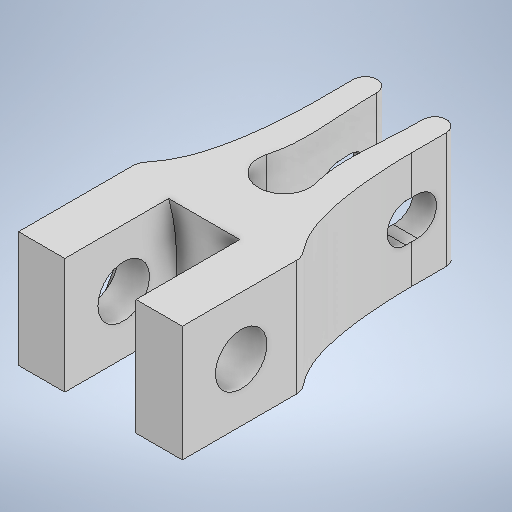
# Autodesk Inventor part: SlideClip
Saved by Autodesk Inventor 2025 (Build 290162010, 162A)
## iProperties
Created: 2025-02-04
Part Number: SlideClip
Material: Generic
Document SubType Name: Modeling
Designer: armenanzasn25
Density: 1 g/cm^3
Appearance: Default
Author: armenanzasn25
Autodesk Inventor part; units mm, degrees
ref_plane "YZ Plane" through (0, 0, 0) normal (1, 0, 0) x (0, 1, 0)
ref_plane "XZ Plane" through (0, 0, 0) normal (0, 1, 0) x (-1, 0, 0)
ref_plane "XY Plane" through (0, 0, 0) normal (0, 0, 1) x (1, 0, 0)
sketch "Sketch1" plane through (0, 0, 0) normal (0, 1, 0) x (-1, 0, 0)
  arc A0 (2.1415, -16.469) -> (0, -13.652) centre (0, -15.8745) ccw
  line L0 (7.0734, 0) -> (7.0734, -9.8745)
  line L1 (0, 0.4443) -> (0, -21.7427) construction
  line L2 (-7.0734, 0) -> (-7.0734, -9.8745)
  arc A1 (0, -13.652) -> (-2.1415, -16.469) centre (0, -15.8745) ccw
  line L3 (4, -22.8384) -> (4, -25.8745)
  line L4 (-4, -22.8384) -> (-4, -25.8745)
  arc A2 (2, -25.8745) -> (4, -25.8745) centre (3, -25.8745) ccw
  arc A3 (-4, -25.8745) -> (-2, -25.8745) centre (-3, -25.8745) ccw
  line L5 (3.0734, 0) -> (3.0734, -9.652)
  line L6 (3.0734, -9.652) -> (-3.0734, -9.652)
  line L7 (-3.0734, -9.652) -> (-3.0734, 0)
  line L8 (7.0734, 0) -> (3.0734, 0)
  line L9 (-3.0734, 0) -> (-7.0734, 0)
  spline S0 degree 4 poles (2, -25.8745) (2, -23.2445) (1.6155, -19.943) (1.6024, -18.411) (2.1415, -16.469) knots 0 0 0 0 0 1 1 1 1 1
  spline S1 degree 4 poles (-2, -25.8745) (-2, -23.2445) (-1.6155, -19.943) (-1.6024, -18.411) (-2.1415, -16.469) knots 0 0 0 0 0 1 1 1 1 1
  spline S2 degree 4 poles (7.0734, -9.8745) (7.0734, -11.5508) (4.5976, -10.8217) (4, -18.7622) (4, -22.8384) knots 0 0 0 0 0 1 1 1 1 1
  spline S3 degree 4 poles (-7.0734, -9.8745) (-7.0734, -11.5508) (-4.5976, -10.8217) (-4, -18.7622) (-4, -22.8384) knots 0 0 0 0 0 1 1 1 1 1
  point P0 (0, 0)
  point P1 (0, -9.652)
  point P2 (1.75, -19.9116)
  point P3 (-1.75, -19.9116)
  point P4 (6.2466, -11.4624)
  point P5 (-6.2466, -11.4624)
  dimension "d6" = 6
  dimension "d7" = 1
  dimension "d8" = 2.2225
  dimension "d19" = 9.652
  dimension "d20" = 6.1468
  dimension "d27" = 4
  dimension "d31" = 4
  dimension "d34" = 3.5
  dimension "d35" = 10
  dimension "d37" = 4
  constraints: 20 end point, 9 symmetric about line, 8 point on circle, 5 perpendicular, 5 vertical, 4 centre point, 2 horizontal alignment, 2 point on line, 1 collinear, 1 horizontal, 1 midpoint, 1 parallel, 1 tangent, 18 other
  measures "d6" vertical distance of L0.end A0.centre
  measures "d7" radius of A2
  measures "d8" radius of A0
  measures "d19" distance of L6.end L7.end
  measures "d20" distance of L5.end L6.end
  measures "d27" distance of point (0, -9.652) A0.end
  measures "d31" distance of L0.start L5.start
  measures "d34" distance of point (-1.75, -19.912) point (1.75, -19.912)
  measures "d35" vertical distance of A0.centre A3.centre
  measures "d37" distance of A3.end A2.start
extrude "Extrusion1" add sketch "Sketch1" along normal blind 10
sketch "Sketch2" plane through (7.0734, 0, 0) normal (1, 0, 0) x (0, 0, -1)
  circle A0 centre (5.08, 5) radius 2.2225
  line L0 (0, 10) -> (9.8745, 10) projected
  line L1 (0, 0) -> (0, 10) projected
  point P0 (9.652, 10)
  dimension "d14" = 4.445
  dimension "d15" = 5
  dimension "d32" = 4.572
  constraints: 1 centre point
  measures "d14" diameter of A0
  measures "d15" distance from line of L0 A0.centre
  measures "d32" horizontal distance of point (9.652, 10) A0.centre
extrude "Extrusion2" cut sketch "Sketch2" against normal blind 15
sketch "Sketch3" plane through (4, 0, -22.8384) normal (1, 0, 0) x (0, 0, -1)
  circle A0 centre (-17.7584, 5) radius 2.2225 projected
  line L0 (3.0361, 0) -> (3.0361, 10) projected
  line L1 (0.0361, 5) -> (1.518, 10) construction
  line L2 (3.0361, 10) -> (0, 10) construction
  line L3 (0.5361, 5) -> (-0.4639, 5) construction
  line L4 (0.5361, 6.651) -> (-0.4639, 6.651)
  line L5 (-0.4639, 3.349) -> (0.5361, 3.349)
  arc A1 (0.5361, 3.349) -> (0.5361, 6.651) centre (0.5361, 5) ccw
  arc A2 (-0.4639, 6.651) -> (-0.4639, 3.349) centre (-0.4639, 5) ccw
  point P0 (-22.8384, 0)
  dimension "d21" = 3
  dimension "d24" = 1
  dimension "d30" = 1.651
  constraints: 10 end point, 4 point on circle, 4 tangent, 2 centre point, 2 midpoint, 1 horizontal, 1 horizontal alignment, 1 parallel
  measures "d21" distance from line of L0 L1.start
  measures "d24" distance of L4.start L4.end
  measures "d30" radius of A2
extrude "Extrusion3" cut sketch "Sketch3" along normal mid plane 20 contours A1 L5 A2 L4
sketch "Sketch4" plane through (-7.0734, 0, -9.8745) normal (-1, 0, 0) x (0, 0, 1)
  line L0 (0, 0) -> (9.8745, 0) projected
  line L1 (9.8745, 0) -> (9.8745, 10) projected
  line L2 (0, 10) -> (9.8745, 10) projected
  line L3 (0, 0) -> (0, 10) projected
  circle A0 centre (4.7945, 5) radius 2.2225 projected
  line L4 (6.9209, 8.683) -> (9.0473, 5)
  line L5 (9.0473, 5) -> (6.9209, 1.317)
  line L6 (6.9209, 1.317) -> (2.6681, 1.317)
  line L7 (2.6681, 1.317) -> (0.5417, 5)
  line L8 (0.5417, 5) -> (2.6681, 8.683)
  line L9 (2.6681, 8.683) -> (6.9209, 8.683)
  dimension "d25" = 7.366
  constraints: 12 end point, 1 coincident, 1 horizontal, 13 other
  measures "d25" distance between parallel lines of L6 L9
extrude "Extrusion4" cut sketch "Sketch4" against normal blind 1.27 contours A0 | L4 L5 L6 L7 L8 L9
sketch "Sketch5" plane through (-4, 0, -25.8745) normal (-1, 0, 0) x (0, 0, 1)
  line L0 (1.3496, 7.921) -> (4.7225, 7.921)
  line L1 (4.7225, 7.921) -> (6.4089, 5)
  line L2 (6.4089, 5) -> (4.7225, 2.079)
  line L3 (4.7225, 2.079) -> (1.3496, 2.079)
  line L4 (1.3496, 2.079) -> (-0.3368, 5)
  line L5 (-0.3368, 5) -> (1.3496, 7.921)
  arc A0 (2.5, 6.651) -> (2.5, 3.349) centre (2.5, 5) ccw projected
  point P0 (25.8745, 0)
  point P1 (3.0361, 5)
  point P2 (3.5, 6.651)
  point P3 (3.5, 3.349)
  point P4 (3.0361, 6.651)
  point P5 (3.0361, 3.349)
  dimension "d38" = 5.842
  constraints: 12 end point, 2 horizontal alignment, 2 vertical alignment, 13 other
  measures "d38" distance between parallel lines of L0 L3
extrude "Extrusion5" cut sketch "Sketch5" along normal mid plane 2.54
sketch "Sketch6" plane through (-3.0734, 0, 0) normal (1, 0, 0) x (0, 0, -1)
  line L0 (9.652, 0) -> (0, 0) projected
  line L1 (9.652, 10) -> (0, 10) projected
  arc A0 (8.9662, 0) -> (8.9662, 10) centre (-8.9178, 5) ccw
  line L2 (0, 10) -> (9.8745, 10) projected
  line L3 (9.8745, 0) -> (9.8745, 10) projected
  line L4 (0, 0) -> (9.8745, 0) projected
  line L5 (9.652, 0) -> (9.652, 10) projected
  point P0 (9.652, 5)
  point P1 (9.652, 4.8706)
  dimension "d41" = 0.6858
  dimension "d44" = 0.6858
  constraints: 2 point on circle, 2 point on line, 1 centre point, 1 tangent
  measures "d41" distance of L1.start A0.end
  measures "d44" distance of L0.start A0.start
extrude "Extrusion6" add sketch "Sketch6" along normal blind 10
equation "\"TUBE\" = 4.445"
equation "\"SCREW\" = 3.302"
equation "\"HEX\" = 5.842"
equation "\"HEX_DEPTH\" = 1.27"
body "Solid1"
